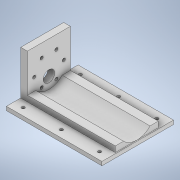
# Autodesk Inventor part: Support_moteur
Saved by Autodesk Inventor 2020.1 (Build 241239000, 239)
## iProperties
Created: 2019-11-14
Part Number: Support_moteur
Material: Generic
Document SubType Name: Modeling
Designer: Admin
Density: 1 g/cm^3
Appearance: Default
Author: Admin
Autodesk Inventor part; units mm, degrees
ref_plane "YZ Plane" through (0, 0, 0) normal (1, 0, 0) x (0, 1, 0)
ref_plane "XZ Plane" through (0, 0, 0) normal (0, 1, 0) x (-1, 0, 0)
ref_plane "XY Plane" through (0, 0, 0) normal (0, 0, 1) x (1, 0, 0)
sketch "Sketch1" plane through (0, 0, 0) normal (0, 0, 1) x (1, 0, 0)
  line L0 (-8.8404, 43.5319) -> (-1.8404, 43.5319)
  line L1 (-1.8404, 43.5319) -> (-1.8404, 3.5319)
  line L2 (-1.8404, 3.5319) -> (90.1596, 3.5319)
  line L3 (90.1596, 3.5319) -> (90.1596, -6.4681)
  line L4 (90.1596, -6.4681) -> (-8.8404, -6.4681)
  line L5 (-8.8404, -6.4681) -> (-8.8404, 43.5319)
  point P0 (0, 0)
  dimension "d0" = 10
  dimension "d1" = 50
  dimension "d2" = 7
  dimension "d4" = 92
  constraints: 12 end point, 4 perpendicular, 2 horizontal
  measures "d0" distance of L2.end L3.end
  measures "d1" distance of L4.end L0.start
  measures "d2" distance of L0.start L0.end
  measures "d4" distance of L1.end L2.end
extrude "Extrusion1" add sketch "Sketch1" along normal blind 45
sketch "Sketch3" plane through (90.1596, -6.4681, 0) normal (1, 0, 0) x (0, 0, -1)
  circle A0 centre (-22.5, 23) radius 19
  line L0 (0, 0) -> (-45, 0) projected
  line L1 (-45, 0) -> (-45, 10) projected
  point P0 (0, 6.4681)
  dimension "d7" = 38
  dimension "d8" = 23
  dimension "d9" = 22.5
  constraints: 1 centre point
  measures "d7" diameter of A0
  measures "d8" distance from line of L0 A0.centre
  measures "d9" distance from line of L1 A0.centre
extrude "Extrusion2" cut sketch "Sketch3" against normal up to surface (92 mm away)
sketch "Sketch4" plane through (-1.8404, 3.5319, 0) normal (1, 0, 0) x (0, 0, -1)
  arc A0 (-36.3564, 0) -> (-8.6436, 0) centre (-22.5, 13) ccw projected
  circle A1 centre (-22.5, 13) radius 19
  circle A2 centre (-22.5, 6) radius 3.25
  line L0 (0, -10) -> (0, 0) projected
  circle A3 centre (-22.5, 13) radius 15.5
  circle A4 centre (-38, 13) radius 2.166
  circle A5 centre (-30.25, 26.4234) radius 2.1809
  circle A6 centre (-14.75, 26.4234) radius 2.0998
  circle A7 centre (-7, 13) radius 1.7963
  circle A8 centre (-14.75, -0.4234) radius 2.628
  circle A9 centre (-30.25, -0.4234) radius 2.0573
  line L1 (-38, 13) -> (-22.5, 13)
  line L2 (-22.5, 13) -> (-7, 13)
  line L3 (-14.75, 26.4234) -> (-22.5, 13)
  line L4 (-14.75, -0.4234) -> (-22.5, 13)
  line L5 (-30.25, -0.4234) -> (-22.5, 13)
  line L6 (-30.25, 26.4234) -> (-22.5, 13)
  point P0 (0, -3.5319)
  dimension "d12" = 38
  dimension "d13" = 7
  dimension "d14" = 6.5
  dimension "d15" = 22.5
  dimension "d16" = 31
  dimension "d17" = 60
  dimension "d18" = 60
  dimension "d19" = 60
  dimension "d20" = 60
  constraints: 12 end point, 9 centre point, 6 point on circle, 2 coincident, 1 collinear, 1 horizontal
  measures "d12" diameter of A1
  measures "d13" distance of A1.centre A2.centre
  measures "d14" diameter of A2
  measures "d15" distance from line of L0 A2.centre
  measures "d16" diameter of A3
  measures "d17" angle of L1 L6
  measures "d18" angle of L6 L3
  measures "d19" angle of L5 L1
  measures "d20" angle of L4 L5
hole "Hole1" at (-1.8404, 29.9553, 30.25) at (-1.8404, 29.9553, 14.75) at (-1.8404, 16.5319, 7) at (-1.8404, 3.1085, 14.75) at (-1.8404, 3.1085, 30.25) at (-1.8404, 16.5319, 38) direction (-1, 0, 0) diameter 3.3 end through all
sketch "Sketch5" plane through (-1.8404, 3.5319, 0) normal (1, 0, 0) x (0, 0, -1)
  point P0 (0, -3.5319)
sketch "Sketch6" plane through (-1.8404, 3.5319, 0) normal (1, 0, 0) x (0, 0, -1)
  circle A0 centre (-22.5, 6) radius 6
  line L0 (-45, 0) -> (-45, 40) projected
  arc A1 (-36.3564, 0) -> (-8.6436, 0) centre (-22.5, 13) ccw projected
  circle A2 centre (-22.5, 13) radius 19
  point P0 (0, -3.5319)
  dimension "d28" = 12
  dimension "d29" = 22.5
  dimension "d30" = 7
  constraints: 2 centre point, 1 coincident
  measures "d28" diameter of A0
  measures "d29" distance from line of L0 A0.centre
  measures "d30" distance of A2.centre A0.centre
extrude "Extrusion3" cut sketch "Sketch6" against normal up to surface (7 mm away) contours A0
sketch "Sketch7" plane through (0, 0, 45) normal (0, 0, 1) x (1, 0, 0)
  line L0 (-8.8404, 43.5319) -> (-8.8404, -6.4681) projected
  line L1 (91.1596, -6.4681) -> (-8.8404, -6.4681)
  line L2 (-8.8404, -6.4681) -> (-8.8404, -2.4681)
  line L3 (-8.8404, -2.4681) -> (91.1596, -2.4681)
  line L4 (91.1596, -2.4681) -> (91.1596, -6.4681)
  point P0 (90.1596, 3.5319)
  dimension "d33" = 4
  dimension "d55" = 100
  constraints: 8 end point, 2 parallel, 1 horizontal, 1 perpendicular, 1 point on line
  measures "d33" distance between parallel lines of L1 L3
  measures "d55" distance of L1.start L1.end
extrude "Extrusion4" add sketch "Sketch7" along normal blind 15 and the other way blind 60
sketch "Sketch8" plane through (-8.8404, -2.4681, 0) normal (0, 1, 0) x (1, 0, 0)
  circle A0 centre (10, 7.5) radius 4.4582
  circle A1 centre (90, 7.5) radius 4.9921
  circle A2 centre (10, -52.5) radius 4.3054
  circle A3 centre (90, -52.5) radius 4.5947
  line L0 (0, 15) -> (100, 15) projected
  line L1 (0, 15) -> (0, 0) projected
  line L2 (100, 15) -> (100, -60) projected
  line L3 (100, 15) -> (100, -60) projected
  line L4 (100, -60) -> (0, -60) projected
  line L5 (0, -45) -> (0, -60) projected
  circle A4 centre (50, -52.5) radius 3.4509
  circle A5 centre (50, 7.5) radius 3.4509
  point P0 (8.8404, 0)
  point P1 (99, 0)
  point P2 (99, -45)
  dimension "d38" = 7.5
  dimension "d39" = 10
  dimension "d40" = 10
  dimension "d41" = 7.5
  dimension "d42" = 10
  dimension "d43" = 7.5
  dimension "d44" = 10
  dimension "d45" = 7.5
  dimension "d53" = 50
  dimension "d54" = 50
  constraints: 6 centre point, 2 other
  measures "d38" distance from line of L0 A0.centre
  measures "d39" distance from line of L1 A0.centre
  measures "d41" distance from line of L0 A1.centre
  measures "d43" distance from line of L4 A3.centre
  measures "d44" distance from line of L5 A2.centre
  measures "d45" distance from line of L4 A2.centre
  measures "d53" distance from line of L1 A5.centre
  measures "d54" distance from line of L5 A4.centre
hole "Hole2" at (1.1596, -2.4681, -7.5) at (81.1596, -2.4681, -7.5) at (81.1596, -2.4681, 52.5) at (1.1596, -2.4681, 52.5) at (41.1596, -2.4681, 52.5) at (41.1596, -2.4681, -7.5) direction (0, -1, 0) diameter 3.3 end through all
body "Solid1"
